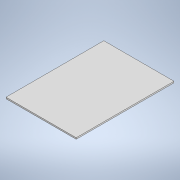
# Autodesk Inventor part: bottom
Saved by Autodesk Inventor 2021 (Build 250183000, 183)
## iProperties
Created: 2020-07-28
Part Number: bottom
Material: Generic
Document SubType Name: Modeling
Designer: johna
Density: 1 g/cm^3
Appearance: Default
Author: johna
Autodesk Inventor part; units mm, degrees
ref_plane "YZ Plane" through (0, 0, 0) normal (1, 0, 0) x (0, 1, 0)
ref_plane "XZ Plane" through (0, 0, 0) normal (0, 1, 0) x (-1, 0, 0)
ref_plane "XY Plane" through (0, 0, 0) normal (0, 0, 1) x (1, 0, 0)
sketch "Sketch1" plane through (0, 0, 0) normal (0, 1, 0) x (-1, 0, 0)
  line L0 (9.4944, 172.6657) -> (-118.1152, 172.6657)
  line L1 (-118.1152, 172.6657) -> (-118.1152, -5.1343)
  line L2 (-118.1152, -5.1343) -> (9.4944, -5.1343)
  line L3 (9.4944, -5.1343) -> (9.4944, 172.6657)
  point P0 (0, 0)
  dimension "d0" = 127.6096
  dimension "d1" = 177.8
  constraints: 8 end point, 2 parallel, 1 horizontal, 1 perpendicular
  measures "d0" distance of L2.end L1.end
  measures "d1" distance of L2.end L0.start
extrude "Extrusion1" add sketch "Sketch1" along normal blind 2.54
body "Solid1"
